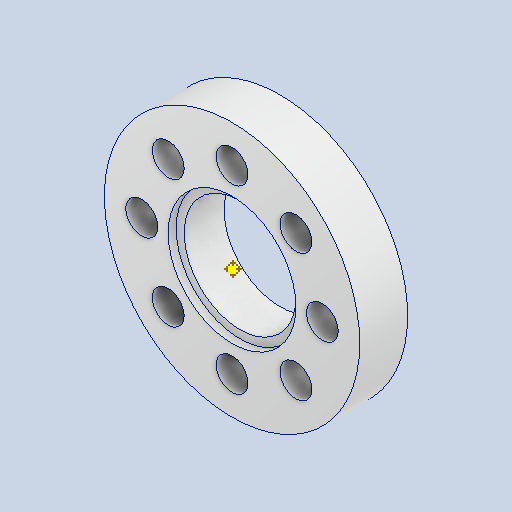
# Autodesk Inventor part: PatternSpacer4mm
Saved by Autodesk Inventor 2023 (Build 270158000, 158)
## iProperties
Created: 2021-01-26
Part Number: PatternSpacer4mm
Material: Aluminum 6061
Document SubType Name: Modeling
Designer: valer
Density: 2.7 g/cm^3
Appearance: Aluminum - Flat
Mass: 8.77918 g
Surface Area: 25.7611 cm^2
Volume: 3.25155 cm^3
Author: valer
Autodesk Inventor part; units mm, degrees
ref_plane "YZ Plane" through (0, 0, 0) normal (1, 0, 0) x (0, 1, 0)
ref_plane "XZ Plane" through (0, 0, 0) normal (0, 1, 0) x (-1, 0, 0)
ref_plane "XY Plane" through (0, 0, 0) normal (0, 0, 1) x (1, 0, 0)
sketch "Base" plane through (0, 0, 0) normal (0, 0, 1) x (1, 0, 0)
  circle A0 centre (0, 0) radius 16
  circle A1 centre (0, 0) radius 7
  circle A2 centre (0, 0) radius 11.3137 construction
  line L0 (-8, 8) -> (8, 8) construction
  line L1 (8, 8) -> (8, -8) construction
  line L2 (8, -8) -> (-8, -8) construction
  line L3 (-8, -8) -> (-8, 8) construction
  circle A3 centre (-8, 8) radius 2
  circle A4 centre (8, 8) radius 2
  circle A5 centre (-8, -8) radius 2
  circle A6 centre (8, -8) radius 2
  circle A7 centre (-11.3137, 0) radius 2
  circle A8 centre (0, 11.3137) radius 2
  line L4 (0, 8) -> (0, -8) construction
  circle A9 centre (11.3137, 0) radius 2
  line L5 (-8, 0) -> (8, 0) construction
  line L6 (0, 11.3137) -> (0, 0) construction
  line L7 (0, 11.3137) -> (0, -8) construction
  line L8 (-11.3137, 0) -> (0, 0) construction
  circle A10 centre (0, -11.3137) radius 2
  line L9 (0, -11.3137) -> (0, 0) construction
  dimension "d0" = 32
  dimension "d1" = 14
  dimension "d2" = 4
  dimension "d3" = 4
  dimension "d4" = 4
  dimension "d5" = 4
  dimension "d6" = 16
  constraints: 20 end point, 10 centre point, 7 coincident, 4 perpendicular, 3 equal radius, 3 midpoint, 2 collinear, 2 horizontal, 2 parallel, 2 symmetric about line, 10 other
  measures "d0" diameter of A0
  measures "d1" diameter of A1
  measures "d2" diameter of A3
  measures "d3" diameter of A4
  measures "d4" diameter of A5
  measures "d5" diameter of A6
  measures "d6" distance of L2.end L0.start
extrude "BaseFeature" add sketch "Base" along normal blind 6
sketch "Indent" plane through (0, 0, 6) normal (0, 0, 1) x (1, 0, 0)
  circle A0 centre (0, 0) radius 8
  dimension "d9" = 16
  constraints: 1 centre point, 1 coincident
  measures "d9" diameter of A0
extrude "IndentFeature" cut sketch "Indent" against normal blind 1
sketch "ShoulderJointPoint" plane through (0, 0, 6) normal (0, 0, 1) x (1, 0, 0)
  point P0 (0, 0)
body "Solid1"
